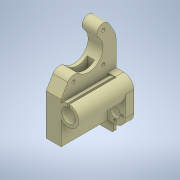
# Autodesk Inventor part: xaxissupport2
Saved by Autodesk Inventor 2020.2 (Build 242310000, 310)
## iProperties
Created: 2017-10-26
Part Number: xaxissupport2
Material: Polipropylen
Document SubType Name: Modeling
Designer: wojte
Density: 0.899 g/cm^3
Appearance: Gładki - popielaty
Author: wojte
Autodesk Inventor part; units mm, degrees
ref_plane "YZ Plane" through (0, 0, 0) normal (1, 0, 0) x (0, 1, 0)
ref_plane "XZ Plane" through (0, 0, 0) normal (0, 1, 0) x (-1, 0, 0)
ref_plane "XY Plane" through (0, 0, 0) normal (0, 0, 1) x (1, 0, 0)
sketch "Szkic1" plane through (0, 0, 0) normal (0, 1, 0) x (-1, 0, 0)
  line L0 (0, 0) -> (16, 0)
  line L1 (16, 0) -> (16, -44)
  line L2 (16, -44) -> (0, -44)
  line L3 (0, -44) -> (0, 0)
  dimension "d0" = 44
  dimension "d1" = 16
  constraints: 8 end point, 2 parallel, 1 horizontal, 1 perpendicular
  measures "d0" distance of L0.end L1.end
  measures "d1" distance of L0.start L0.end
extrude "Wyciągnięcie proste1" add sketch "Szkic1" along normal blind 59
sketch "Szkic2" plane through (0, 59, 0) normal (0, 1, 0) x (1, 0, 0)
  line L0 (0, 44) -> (19, 44)
  line L1 (19, 44) -> (19, 0)
  line L2 (19, 0) -> (0, 0)
  line L3 (0, 0) -> (0, 44)
  dimension "d4" = 19
  constraints: 8 end point, 2 parallel, 2 point on line, 1 coincident, 1 horizontal, 1 perpendicular
  measures "d4" distance of L0.start L0.end
extrude "Wyciągnięcie proste2" add sketch "Szkic2" against normal blind 9
fillet "Zaokrąglenie1" radius 11 2 edges at (19, 54.5, 0) (19, 54.5, -44)
sketch "Szkic3" plane through (0, 59, 0) normal (0, 1, 0) x (1, 0, 0)
  arc A0 (8, 0) -> (19, 11) centre (8, 11) ccw projected
  point P0 (0, 0)
  constraints: 1 coincident
hole "Otwór1" at (8, 59, -11) direction (0, -1, 0) diameter 15 end through all
sketch "Szkic4" plane through (0, 59, 0) normal (0, 1, 0) x (1, 0, 0)
  arc A0 (19, 33) -> (8, 44) centre (8, 33) ccw projected
  point P0 (0, 0)
  point P1 (8, 32.5)
  dimension "d85" = 0.5
  constraints: 1 vertical alignment
  measures "d85" distance of A0.centre point (8, 32.5)
hole "Otwór2" at (8, 59, -32.5) direction (0, -1, 0) diameter 11 end through all
sketch "Szkic5" plane through (0, 59, 0) normal (0, 1, 0) x (1, 0, 0)
  circle A0 centre (8, 32.5) radius 5.5 projected
  point P0 (0, 0)
  point P1 (8, 24.5)
  point P2 (16, 32.5)
  point P3 (8, 40.5)
  point P4 (0, 32.5)
  dimension "d23" = 8
  dimension "d26" = 360
  constraints: 1 vertical alignment, 5 other
  measures "d23" distance of A0.centre point (8, 24.5)
hole "Otwór3" at (8, 59, -24.5) at (16, 59, -32.5) at (8, 59, -40.5) at (0, 59, -32.5) direction (0, -1, 0) diameter 3 depth 9 tip angle 118
sketch "Szkic6" plane through (0, 50, 0) normal (0, -1, 0) x (1, 0, 0)
  arc A0 (19, -11) -> (8, 0) centre (8, -11) ccw projected
  arc A1 (7, -0.0455) -> (9, -0.0455) centre (8, -11) ccw
  line L0 (8, -11) -> (8, 0) construction
  line L1 (9, -3.567) -> (9, 0)
  line L2 (7, -3.567) -> (7, 0)
  circle A2 centre (8, -11) radius 7.5 projected
  point P0 (0, 0)
  dimension "d35" = 22
  dimension "d36" = 2
  constraints: 6 end point, 4 point on circle, 2 parallel, 2 point on line, 1 centre point, 1 coincident, 1 vertical, 1 other
  measures "d35" diameter of A1
  measures "d36" distance between parallel lines of L2 L1
extrude "Wyciągnięcie proste3" add sketch "Szkic6" along normal up to surface (50 mm away) contours A1 L2 A2 L1 A0
sketch "Szkic7" plane through (0, 59, 0) normal (0, 1, 0) x (1, 0, 0)
  line L0 (0, 3.4502) -> (0, 0) projected
  line L1 (0, 0) -> (-16, 0)
  line L2 (-16, 0) -> (-16, -52)
  line L3 (-16, -52) -> (0, -52)
  line L4 (0, -52) -> (0, 0)
  dimension "d39" = 52
  constraints: 8 end point, 2 parallel, 1 coincident, 1 horizontal, 1 perpendicular
  measures "d39" distance of L1.end L2.end
extrude "Wyciągnięcie proste4" add sketch "Szkic7" against normal up to surface (59 mm away)
sketch "Szkic8" plane through (0, 50, 0) normal (1, 0, 0) x (0, 0, -1)
  line L0 (-52, 9) -> (-52, -50) projected
  line L1 (-52, -20.5) -> (-26, -20.5) construction
  line L2 (-52, 9) -> (0, 9) projected
  point P0 (0, -50)
  dimension "d94" = 26
  constraints: 2 end point, 1 coincident, 1 horizontal, 1 midpoint
  measures "d94" distance from line of L0 point (-26, -20.5)
hole "Otwór4" at (0, 29.5, 26) direction (-1, 0, 0) diameter 31 end through all
sketch "Szkic9" plane through (0, 50, 0) normal (1, 0, 0) x (0, 0, -1)
  circle A0 centre (-26, -20.5) radius 15.5 projected
  line L0 (-52, 9) -> (-52, -50) projected
  line L1 (3.4502, -50) -> (-52, -50) projected
  point P0 (0, -50)
  point P1 (-41.75, -4.75)
  point P2 (-9.75, -36.75)
  point P3 (-9.75, -4.75)
  dimension "d52" = 32
  dimension "d53" = 32
  dimension "d95" = 10.25
  dimension "d96" = 13.25
  constraints: 1 horizontal alignment, 1 vertical alignment
  measures "d52" distance of point (-9.75, -4.75) point (-41.75, -4.75)
  measures "d53" distance of point (-9.75, -36.75) point (-9.75, -4.75)
  measures "d95" distance from line of L0 point (-41.75, -4.75)
  measures "d96" distance from line of L1 point (-9.75, -36.75)
hole "Otwór5" at (0, 45.25, 41.75) at (0, 13.25, 9.75) at (0, 45.25, 9.75) direction (-1, 0, 0) diameter 3.4 end through all
sketch "Szkic10" plane through (0, 50, 0) normal (1, 0, 0) x (0, 0, -1)
  line L0 (0, -50) -> (-12.307, -42.8945)
  arc A0 (-14.3302, -30.7012) -> (-12.307, -42.8945) centre (-8.307, -35.9663) ccw
  line L1 (3.4502, -50) -> (-52, -50) projected
  circle A1 centre (-41.75, -4.75) radius 1.7 projected
  arc A2 (-45.1369, 1.1163) -> (-36.9602, -9.5398) centre (-41.75, -4.75) ccw
  line L2 (-45.1369, 1.1163) -> (-31.482, 9)
  line L3 (44, 9) -> (-52, 9) projected
  arc A3 (-36.9602, -9.5398) -> (-14.3302, -30.7012) centre (-26, -20.5) ccw
  circle A4 centre (-26, -20.5) radius 15.5 projected
  line L4 (-31.482, 9) -> (-52, 9)
  line L5 (-52, 9) -> (-52, -50) projected
  line L6 (-52, -50) -> (0, -50)
  line L7 (-52, 9) -> (-52, -50)
  dimension "d61" = 30
  dimension "d62" = 8
  dimension "d63" = 31
  dimension "d64" = 30
  constraints: 10 end point, 6 point on circle, 4 tangent, 3 centre point, 2 coincident, 2 collinear, 1 perpendicular, 1 point on line
  measures "d61" angle of L1 L0
  measures "d62" radius of A0
  measures "d63" diameter of A3
  measures "d64" angle of L3 L2
extrude "Wyciągnięcie proste5" cut sketch "Szkic10" against normal through all contours L1 L5 L3 L2 A2 A3 A0 L0
fillet "Zaokrąglenie2" radius 20 1 edges at (-8, 59, 31.482)
sketch "Szkic11" plane through (0, 0, -44) normal (0, 0, -1) x (-1, 0, 0)
  line L0 (12, 19) -> (4, 19)
  line L1 (4, 19) -> (4, 40)
  line L2 (4, 40) -> (12, 40)
  line L3 (12, 40) -> (12, 19)
  line L4 (-8, 59) -> (16, 59) projected
  line L5 (0, 0) -> (16, 0) projected
  line L6 (8, 0) -> (8, 59) construction
  dimension "d68" = 8
  dimension "d69" = 21
  dimension "d70" = 19
  constraints: 10 end point, 2 parallel, 1 horizontal, 1 midpoint, 1 perpendicular, 1 point on line, 1 vertical, 1 other
  measures "d68" distance of L1.end L2.end
  measures "d69" distance of L0.end L1.end
  measures "d70" distance between parallel lines of L4 L2
extrude "Wyciągnięcie proste6" cut sketch "Szkic11" against normal up to surface
sketch "Szkic12" plane through (0, 0, -44) normal (0, 0, -1) x (-1, 0, 0)
  line L0 (4, 19) -> (4, 40) projected
  line L1 (12, 40) -> (12, 19) projected
  line L2 (0, 0) -> (0, 50) projected
  line L3 (-8, 59) -> (16, 59) projected
  line L4 (4, 40) -> (12, 40) projected
  line L5 (12, 19) -> (4, 19) projected
  point P0 (8, 52)
  point P1 (8, 7)
  dimension "d73" = 8
  dimension "d76" = 12
  dimension "d77" = 12
  constraints: 1 vertical alignment
  measures "d73" distance from line of point (8, 52) L2
  measures "d76" distance from line of L4 point (8, 52)
  measures "d77" distance from line of L5 point (8, 7)
hole "Otwór6" at (-8, 52, -44) at (-8, 7, -44) direction (0, 0, 1) diameter 8 depth 35 tip angle 118
thread "Gwint1" size "M3.5x0.6" class "6H" standard "ANSI Metric M Profile" full length
thread "Gwint2" size "M3.5x0.6" class "6H" standard "ANSI Metric M Profile" full length
thread "Gwint3" size "M3.5x0.6" class "6H" standard "ANSI Metric M Profile" full length
thread "Gwint4" size "M3.5x0.6" class "6H" standard "ANSI Metric M Profile" full length
sketch "Szkic13" plane through (0, 0, -44) normal (0, 0, -1) x (-1, 0, 0)
  line L0 (-8, 59) -> (16, 59) projected
  line L1 (16, 56.3205) -> (0, 56.3205) projected
  line L2 (16, 59) -> (0, 59)
  line L3 (0, 59) -> (0, 56.3205)
  line L4 (0, 56.3205) -> (16, 56.3205)
  line L5 (16, 56.3205) -> (16, 59)
  point P0 (0, 0)
  constraints: 8 end point, 2 parallel, 1 horizontal, 1 perpendicular
extrude "Wyciągnięcie proste7" add sketch "Szkic13" along normal blind 15
sketch "Szkic14" plane through (0, 59, 0) normal (0, 1, 0) x (1, 0, 0)
  line L0 (-16, 59) -> (0, 59) projected
  line L1 (-8, 59) -> (-8, -26.123) construction
  line L2 (0, -26.123) -> (-16, -26.123) projected
  point P0 (0, 0)
  point P1 (-12.75, 51.5)
  point P2 (-3.25, 51.5)
  dimension "d99" = 9.5
  dimension "d100" = 7.5
  constraints: 2 end point, 2 midpoint, 1 horizontal alignment, 1 symmetric about line
  measures "d99" distance of point (-3.25, 51.5) point (-12.75, 51.5)
  measures "d100" distance from line of L0 point (-12.75, 51.5)
hole "Otwór7" at (-12.75, 59, -51.5) at (-3.25, 59, -51.5) direction (0, -1, 0) diameter 2 end through all
fillet "Zaokrąglenie3" radius 2 3 edges at (0, 57.6603, -59) (-16, 57.6603, -59) (0, 57.6603, -44)
